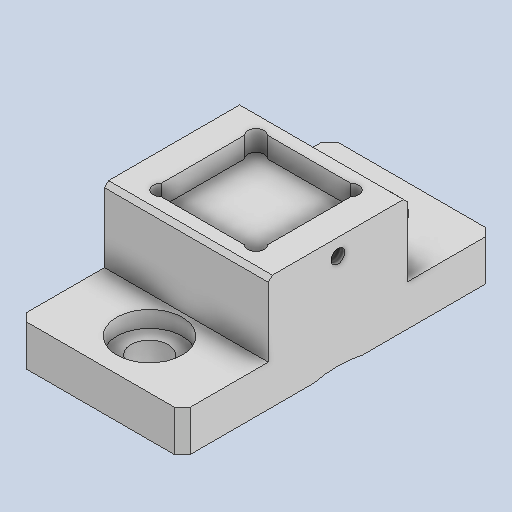
# Autodesk Inventor part: ADAPTER_PBS-BH19.05-CS12.7
Saved by Autodesk Inventor 2024.2 (Build 282272000, 272)
## iProperties
Created: 2020-10-22
Part Number: ADAPTER_PBS-BH19.05-CS12.7
Material: Generic
Document SubType Name: Modeling
Designer: qiti1
Density: 1 g/cm^3
Appearance: Default
ItemSpecifications: {"_id":"6046923b8c5dc80009334eb8","finish":"543ef1f380da5b0c476373c1","finish_location":null,"material":"5515e170db035c20ce34af9a","process_initialism":null,"quotes":null,"current_quote":null,"quantity_ordered":50,"features":null,"hardware":null,"threading":{"quantity":1},"part_markings":[],"surface_roughness":null,"tolerance":null,"weld_quantity":null,"Notes":" :: Thread Spec: 1x See Notes/Drawing :: \r\n","certifications":[],"part":null,"revision_num":0,"last_history":null,"inspection_requirement_details":{"inspection_requirement":"std","customer_data_sheet":null},"feedback":null}
Author: qiti1
Autodesk Inventor part; units mm, degrees
ref_plane "YZ Plane" through (0, 0, 0) normal (1, 0, 0) x (0, 1, 0)
ref_plane "XZ Plane" through (0, 0, 0) normal (0, 1, 0) x (-1, 0, 0)
ref_plane "XY Plane" through (0, 0, 0) normal (0, 0, 1) x (1, 0, 0)
sketch "Sketch1" plane through (0, 0, 0) normal (0, 1, 0) x (-1, 0, 0)
  line L0 (10, 8.5) -> (-10, 8.5)
  line L1 (-10, 8.5) -> (-10, -8.5)
  line L2 (-10, -8.5) -> (10, -8.5)
  line L3 (10, -8.5) -> (10, 8.5)
  line L4 (10, 8.5) -> (-10, -8.5) construction
  line L5 (-10, 8.5) -> (10, -8.5) construction
  point P0 (0, 0)
  dimension "POST_WIDTH" = 17
  dimension "POST_LENGTH" = 20
  constraints: 12 end point, 2 midpoint, 2 parallel, 1 horizontal, 1 perpendicular
  measures "POST_WIDTH" distance of L2.end L0.start
  measures "POST_LENGTH" distance of L1.end L2.end
extrude "Extrusion1" add sketch "Sketch1" along normal blind 11.45
sketch "Sketch2" plane through (0, 0, 0) normal (0, -1, 0) x (1, 0, 0)
  line L0 (-10, -19) -> (10, -19)
  line L1 (10, -19) -> (10, 19)
  line L2 (10, 19) -> (-10, 19)
  line L3 (-10, 19) -> (-10, -19)
  line L4 (-10, -19) -> (10, 19) construction
  line L5 (10, -19) -> (-10, 19) construction
  line L6 (-10, -8.5) -> (-10, 8.5) projected
  line L7 (-10, 8.5) -> (10, 8.5) projected
  point P0 (0, 0)
  dimension "d4" = 0
  dimension "d5" = 10.5
  constraints: 12 end point, 2 midpoint, 2 parallel, 1 horizontal, 1 perpendicular
  measures "d4" distance between parallel lines of L6 L3
  measures "d5" distance between parallel lines of L2 L7
extrude "Extrusion2" add sketch "Sketch2" against normal blind 5
chamfer "Chamfer6" distance 1 angle 45 4 edges at (10, 2.5, 19) (-10, 2.5, 19) (10, 2.5, -19) (-10, 2.5, -19)
sketch "Sketch3" plane through (0, 5, 0) normal (0, 1, 0) x (1, 0, 0)
  line L0 (-10, 19) -> (10, 19) projected
  line L1 (0, 19) -> (0, -19)
  line L2 (10, -19) -> (-10, -19) projected
  line L3 (10, -8.5) -> (10, 8.5) projected
  line L4 (10, 0) -> (-10, 0)
  line L5 (-10, -19) -> (-10, 19) projected
  point P0 (0, 0)
  point P1 (0, -13)
  point P2 (0, 13)
  dimension "d15" = 0
  dimension "d16" = 6
  constraints: 4 end point, 4 midpoint, 1 symmetric about line
  measures "d15" distance from line of L1 point (0, -13)
  measures "d16" distance from line of L2 point (0, -13)
hole "Hole1" at (0, 5, 13) at (0, 5, -13) direction (0, -1, 0) diameter 4.5 end through all counterbore diameter 8 counterbore depth 2 clearance for "Socket Head Cap Screw" size "#8" standard "Ansi Unified Screw Threads"
sketch "Sketch10" plane through (0, 11.45, 0) normal (0, 1, 0) x (1, 0, 0)
  line L0 (-6.5, 6.5) -> (6.5, 6.5)
  line L1 (6.5, 6.5) -> (6.5, -6.5)
  line L2 (6.5, -6.5) -> (-6.5, -6.5)
  line L3 (-6.5, -6.5) -> (-6.5, 6.5)
  line L4 (-6.5, 6.5) -> (6.5, -6.5) construction
  line L5 (6.5, 6.5) -> (-6.5, -6.5) construction
  line L6 (-10, 8.5) -> (-10, -8.5) projected
  line L7 (10, 8.5) -> (-10, 8.5) projected
  line L8 (10, 8.5) -> (10, -8.5) projected
  line L9 (10, -8.5) -> (-10, -8.5)
  line L10 (-10, -8.5) -> (-10, 8.5)
  line L11 (-10, 8.5) -> (10, 8.5)
  line L12 (10, 8.5) -> (10, -8.5)
  circle A0 centre (5.7929, 5.7929) radius 1
  circle A1 centre (5.7929, -5.7929) radius 1
  circle A2 centre (-5.7929, -5.7929) radius 1
  circle A3 centre (-5.7929, 5.7929) radius 1
  point P0 (0, 0)
  point P1 (0, 0)
  point P2 (10, -18)
  point P3 (-10, -8.5)
  point P4 (-6.5, 5.0858)
  point P5 (-5.0858, 6.5)
  point P6 (5.0858, 6.5)
  point P7 (6.5, 5.0858)
  point P8 (6.5, -5.0858)
  point P9 (5.0858, -6.5)
  point P10 (-5.0858, -6.5)
  point P11 (-6.5, -5.0858)
  dimension "d173" = 2
  dimension "d174" = 2
  dimension "d175" = 2
  dimension "d176" = 2
  dimension "d66" = 10
  dimension "d67" = 8.5
  dimension "CUBE_GROOVE_LENGTH" = 13
  dimension "CUBE_GROOVE_WIDTH" = 13
  constraints: 20 end point, 4 parallel, 4 point on line, 2 horizontal, 2 midpoint, 2 perpendicular, 12 other
  measures "d66" distance from line of L6 point (0, 0)
  measures "d67" distance from line of L7 point (0, 0)
  measures "CUBE_GROOVE_LENGTH" distance between parallel lines of L3 L1
  measures "CUBE_GROOVE_WIDTH" distance between parallel lines of L2 L0
extrude "Extrusion8" add sketch "Sketch10" along normal blind 2.5
chamfer "Chamfer4" distance 0.5 angle 45 2 edges at (0, 13.95, 8.5) (0, 13.95, -8.5)
sketch "Sketch13" plane through (10, 0, 18) normal (1, 0, 0) x (0, 0, -1)
  line L0 (26.5, 5) -> (26.5, 13.45) projected
  line L1 (10, 13.95) -> (26, 13.95) projected
  point P0 (18, 0)
  point P1 (18, 11.95)
  dimension "d132" = 8.5
  dimension "d177" = 2
  measures "d132" distance from line of L0 point (18, 11.95)
  measures "d177" distance from line of point (18, 11.95) L1
hole "Hole6" at (10, 11.95, 0) direction (-1, 0, 0) diameter 1.6942 depth 3.5 thread size "2-56 UNC" class "2B" standard "ANSI Unified Screw Threads"
sketch "Sketch14" plane through (0, 11.45, 0) normal (0, 1, 0) x (1, 0, 0)
  line L0 (5.5, -3) -> (5.5, 3) construction
  line L1 (6.5, -3) -> (6.5, 3)
  line L2 (4.5, 3) -> (4.5, -3)
  arc A0 (4.5, -3) -> (6.5, -3) centre (5.5, -3) ccw
  arc A1 (6.5, 3) -> (4.5, 3) centre (5.5, 3) ccw
  line L3 (6.5, 5.0858) -> (6.5, -5.0858) projected
  point P0 (0, 0)
  point P1 (5.5, 0)
  point P2 (6.5, 4.7679)
  point P3 (6.5, -4.7679)
  point P4 (6.5, 5.5)
  point P5 (6.5, -5.5)
  dimension "d134" = 0
  dimension "d136" = 3
  dimension "d137" = 1
  dimension "d138" = 0
  constraints: 8 end point, 4 point on circle, 4 tangent, 2 centre point, 1 midpoint, 1 parallel, 1 vertical
  measures "d134" distance between parallel lines of L1 L3
  measures "d136" distance of point (5.5, 0) L0.end
  measures "d137" radius of A1
  measures "d138" vertical distance of point (0, 0) point (5.5, 0)
extrude "Extrusion9" cut sketch "Sketch14" against normal blind 1
sketch "Sketch15" plane through (0, 0, 0) normal (0, -1, 0) x (1, 0, 0)
  line L0 (0, -4.5) -> (0, -5.5) construction
  line L1 (-1.05, -4.5) -> (-1.05, -5.5)
  line L2 (1.05, -5.5) -> (1.05, -4.5)
  arc A0 (1.05, -4.5) -> (-1.05, -4.5) centre (0, -4.5) ccw
  arc A1 (-1.05, -5.5) -> (1.05, -5.5) centre (0, -5.5) ccw
  point P0 (0, 0)
  point P1 (0, 5)
  point P2 (0, -5)
  dimension "d162" = 0
  dimension "d163" = 0
  dimension "d164" = 10
  dimension "d165" = 5
  dimension "d166" = 1
  dimension "d167" = 1.05
  constraints: 8 end point, 4 point on circle, 4 tangent, 2 centre point, 1 midpoint, 1 parallel, 1 vertical
  measures "d162" horizontal distance of point (0, -5) point (0, 5)
  measures "d163" horizontal distance of point (0, 0) point (0, -5)
  measures "d164" distance of point (0, -5) point (0, 5)
  measures "d165" distance of point (0, -5) point (0, 0)
  measures "d166" distance of L0.start L0.end
  measures "d167" radius of A1
hole "Hole7" at (0, 0, 5) direction (0, 1, 0) diameter 2.1 depth 2.1
extrude "Extrusion10" cut sketch "Sketch15" against normal blind 2.1
sketch "Sketch16" plane through (10, 0, 18) normal (1, 0, 0) x (0, 0, -1)
  circle A0 centre (18, -12.35) radius 12.7
  point P0 (18, 0)
  dimension "d168" = 0
  dimension "d169" = 25.4
  dimension "d170" = 12.35
  constraints: 1 centre point
  measures "d168" horizontal distance of A0.centre point (18, 0)
  measures "d169" diameter of A0
  measures "d170" distance of point (18, 0) A0.centre
extrude "Extrusion11" cut sketch "Sketch16" against normal up to surface (20 mm away)
equation "\"d66\" = 0.5 * POST_LENGTH"
equation "\"d67\" = 0.5 * POST_WIDTH"
equation "\"CUBE_GROOVE_LENGTH\" = CUBE_SIZE + CUBE_GROVE_GAP"
equation "\"CUBE_GROOVE_WIDTH\" = CUBE_SIZE + CUBE_GROVE_GAP"
equation "\"d132\" = 0.5 * POST_WIDTH"
equation "\"BEAM_HEIGHT\" = 19.05"
equation "\"CUBE_SIZE\" = 12.7"
equation "\"CUBE_GROVE_GAP\" = 0.3"
body "Solid1"
